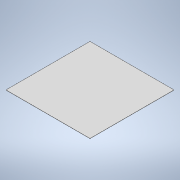
# Autodesk Inventor part: electrode
Saved by Autodesk Inventor 2021 (Build 250183000, 183)
## iProperties
Created: 2020-07-14
Part Number: electrode
Material: Generic
Document SubType Name: Modeling
Designer: aydan
Density: 1 g/cm^3
Appearance: Default
Author: aydan
Autodesk Inventor part; units mm, degrees
ref_plane "YZ Plane" through (0, 0, 0) normal (1, 0, 0) x (0, 1, 0)
ref_plane "XZ Plane" through (0, 0, 0) normal (0, 1, 0) x (-1, 0, 0)
ref_plane "XY Plane" through (0, 0, 0) normal (0, 0, 1) x (1, 0, 0)
sketch "Sketch1" plane through (0, 0, 0) normal (0, 1, 0) x (-1, 0, 0)
  line L0 (23, 23) -> (-23, 23)
  line L1 (-23, 23) -> (-23, -23)
  line L2 (-23, -23) -> (23, -23)
  line L3 (23, -23) -> (23, 23)
  line L4 (23, 23) -> (-23, -23) construction
  line L5 (-23, 23) -> (23, -23) construction
  point P0 (0, 0)
  dimension "d0" = 46
  dimension "d1" = 46
  constraints: 12 end point, 2 midpoint, 2 parallel, 1 horizontal, 1 perpendicular
  measures "d0" distance of L2.end L1.end
  measures "d1" distance of L1.end L0.end
extrude "Extrusion1" add sketch "Sketch1" along normal blind 0.1
body "Solid1"
